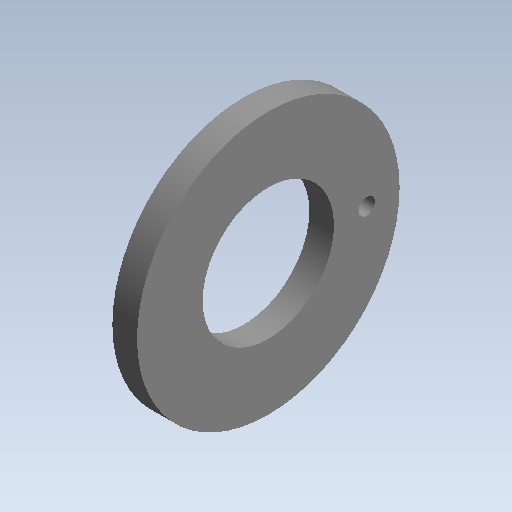
# Autodesk Inventor part: LFW-0815
Saved by Autodesk Inventor 2020.4 (Build 244396000, 396)
## iProperties
Part Number: LFW-0815
Material: 一般
Catalog Web Link: www.cadenas.de
Description: 既製品
Vendor: OILES
Document SubType Name: Modeling
Designer: partserver
Manufacturer: OILES
Mass: 0.225017 g
Surface Area: 4.17832 cm^2
Volume: 0.225017 cm^3
Density: 1 g/cm^3
Appearance: PSOLRGB-175-175-175
Category: PARTsolutions
Company: OILES
PSOL_IDENT_0: {$CADENAS_DATA\23d-libs\oiles\multi_bearings\oiles_drymet_lf\washer_lfw.prj},157 {VTYP=3D},{NB=LFW-0
PSOL_IDENT_1: 815},{LINA=LFW-0815},{NN=Washers},{DATE=15.04.2019 22:54:28},{GEOMDATE=27.10.2016 04:18:17},{VERSION=
PSOL_IDENT_2: },{LINEID=10},{WBVAR=},{WBNUMERIC=}  {NB=LFW-0815},{LINA=LFW-0815},{KT=DUMMY},{ORDERNO=LFW-0815},{ID=
PSOL_IDENT_3: 8},{IDT=+0.25/0},{OD=16},{ODT=0/-0.25},{T=1.5},{TT=-0.03/-0.08},{KPH=1.0},{KHT=+0.30/+0.10},{PCD=12}
PSOL_IDENT_4: ,{PDT=±0.12},{TE=-200~+280°C},{P=49.0N/mm2 (500kgf/cm2)},{V=0.65m/s (39m/min)},{PV=3.60N/mm2•m/s  (2
PSOL_IDENT_5: ,200kgf/cm2•m/min)},{CAU=Please refer to catalog about detail.}
NB: LFW-0815
NN: Washers
NT: LFW
NBSYN: $ORDERNO.
LINA: LFW-0815
CATALOG: OILES CORPORATION
ORDERNO: LFW-0815
ID: 8
IDT: +0.25/0
OD: 16
ODT: 0/-0.25
T: 1.5
TT: -0.03/-0.08
KPH: 1
KHT: +0.30/+0.10
PCD: 12
PDT: ±0.12
TE: -200~+280°C
P: 49.0N/mm2 (500kgf/cm2)
V: 0.65m/s (39m/min)
PV: 3.60N/mm2•m/s  (2,200kgf/cm2•m/min)
CAU: Please refer to catalog about detail.
SUPPLIER: OILES
ARTICLENO: LFW-0815
BOMINFO: LFW-0815
CREATOR: CADENAS GmbH
Title: LFW-0815
Author: Cadenas PARTsolutions
Comments: LFW
Autodesk Inventor part; units mm, degrees
ref_plane "YZ Plane" through (0, 0, 0) normal (1, 0, 0) x (0, 1, 0)
ref_plane "XZ Plane" through (0, 0, 0) normal (0, 1, 0) x (-1, 0, 0)
ref_plane "XY Plane" through (0, 0, 0) normal (0, 0, 1) x (1, 0, 0)
sketch "Sketch_1" plane through (0, 0, 0) normal (0, 0, 1) x (1, 0, 0)
  line L0 (1.5, 0) -> (0, 0)
  line L1 (0, 4) -> (1.5, 4)
  line L2 (1.5, 4) -> (1.5, 8)
  line L3 (1.5, 8) -> (0, 8)
  line L4 (0, 8) -> (0, 4)
  constraints: 10 end point
revolve "Revolution1" add sketch "Sketch_1" angle 360 about axis through (1.5, 0, 0) along (1, 0, 0)
sketch "Sketch2" plane through (1.5, 0, 0) normal (1, 0, 0) x (0, 0, -1)
  point P0 (0, 6)
hole "Hole1" at (1.5, 6, 0) direction (-1, 0, 0) diameter 1 depth 1.5
body "Solid1"
